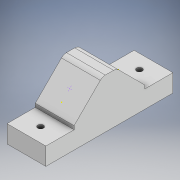
# Autodesk Inventor part: StrutConnector
Saved by Autodesk Inventor 2022 (Build 260153000, 153)
## iProperties
Created: 2021-05-06
Part Number: StrutConnector
Material: Generic
Document SubType Name: Modeling
Designer: Mick Veldhuis
Density: 1 g/cm^3
Appearance: Default
Author: Mick Veldhuis
Autodesk Inventor part; units mm, degrees
ref_plane "YZ Plane" through (0, 0, 0) normal (1, 0, 0) x (0, 1, 0)
ref_plane "XZ Plane" through (0, 0, 0) normal (0, 1, 0) x (-1, 0, 0)
ref_plane "XY Plane" through (0, 0, 0) normal (0, 0, 1) x (1, 0, 0)
sketch "Sketch1" plane through (0, 0, 0) normal (0, 1, 0) x (-1, 0, 0)
  line L0 (11, 36) -> (-11, 36)
  line L1 (-11, 36) -> (-11, -36)
  line L2 (-11, -36) -> (11, -36)
  line L3 (11, -36) -> (11, 36)
  line L4 (11, 36) -> (-11, -36) construction
  line L5 (-11, 36) -> (11, -36) construction
  point P0 (0, 0)
  constraints: 12 end point, 2 midpoint, 2 parallel, 1 horizontal, 1 perpendicular
extrude "Extrusion1" add sketch "Sketch1" along normal blind 10
sketch "Sketch2" plane through (0, 10, 0) normal (0, 1, 0) x (1, 0, 0)
  point P0 (0, 0)
  point P1 (0, -28)
  point P2 (0, 28)
hole "Hole1" at (0, 10, 28) at (0, 10, -28) direction (0, -1, 0) diameter 3.242 depth 10 thread size "M4x0.7" class "6H" standard "ISO Metric profile"
sketch "Sketch3" plane through (0, 10, 0) normal (0, 1, 0) x (1, 0, 0)
  line L0 (11, -36) -> (11, 36) projected
  line L1 (-11, -20) -> (11, -20)
  line L2 (11, -20) -> (11, 20)
  line L3 (11, 20) -> (-11, 20)
  line L4 (-11, 20) -> (-11, -20)
  line L5 (-11, -20) -> (11, 20) construction
  line L6 (11, -20) -> (-11, 20) construction
  point P0 (0, 0)
  constraints: 12 end point, 2 midpoint, 2 parallel, 1 horizontal, 1 perpendicular, 1 point on line
extrude "Extrusion2" add sketch "Sketch3" along normal blind 18
chamfer "Chamfer1" distance 16 angle 45 2 edges at (0, 28, -20) (0, 28, 20)
fillet "Fillet1" radius 4 2 edges at (0, 28, 4) (0, 28, -4)
sketch "Sketch4" plane through (-11, 12, 20) normal (0, 0.7071, 0.7071) x (1, 0, 0)
  point P0 (11, 5.6569)
  point P1 (11, 12)
sketch "Sketch5" plane through (11, 12, -20) normal (0, 0.7071, -0.7071) x (-1, 0, 0)
  point P0 (11, 5.6569)
  point P1 (11, 12)
body "Solid1"
